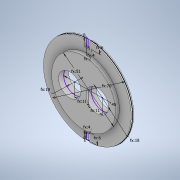
# Autodesk Inventor part: Spacer
Saved by Autodesk Inventor 2021.2 (Build 252289000, 289)
## iProperties
Created: 2023-01-29
Part Number: Spacer
Material: Типовые
Document SubType Name: Modeling
Designer: Andrei
Density: 1 g/cm^3
Appearance: По умолчанию
Author: Andrei
Autodesk Inventor part; units mm, degrees
ref_plane "YZ Plane" through (0, 0, 0) normal (1, 0, 0) x (0, 1, 0)
ref_plane "XZ Plane" through (0, 0, 0) normal (0, 1, 0) x (-1, 0, 0)
ref_plane "XY Plane" through (0, 0, 0) normal (0, 0, 1) x (1, 0, 0)
sketch "Эскиз1" plane through (0, 0, 0) normal (0, 0, 1) x (1, 0, 0)
  circle A0 centre (0, 0) radius 35
  circle A1 centre (0, 0) radius 25.5
  circle A2 centre (11, 0) radius 9
  circle A3 centre (-11, 0) radius 9
  line L0 (-2.0313, 35) -> (1.9687, 35)
  line L1 (1.9687, 35) -> (1.9687, 29)
  line L2 (1.9687, 29) -> (-2.0313, 29)
  line L3 (-2.0313, 29) -> (-2.0313, 35)
  line L4 (-2.0313, -29) -> (1.9687, -29)
  line L5 (1.9687, -29) -> (1.9687, -35)
  line L6 (1.9687, -35) -> (-2.0313, -35)
  line L7 (-2.0313, -35) -> (-2.0313, -29)
  line L8 (-0.0313, 25.5) -> (-0.0313, -25.5)
  line L9 (-0.0313, -25.5) -> (-0.0313, -35)
  line L10 (-0.0313, 35) -> (-0.0313, 25.5)
  point P0 (-2.0313, 25.419)
  point P1 (-2.0313, -25.419)
  point P2 (1.9687, -25.4239)
  point P3 (1.9687, 25.4239)
  point P4 (1.9687, -34.9446)
  point P5 (1.9687, 34.9446)
  point P6 (-2.0313, 34.941)
  point P7 (-2.0313, -34.941)
  dimension "d0" = 70
  dimension "d1" = 51
  dimension "d2" = 18
  dimension "d3" = 18
  dimension "d4" = 11
  dimension "d5" = 11
  dimension "d6" = 40
  dimension "d7" = 4
  dimension "d8" = 4
  dimension "d9" = 6
  dimension "d10" = 6
  dimension "d11" = 2
  dimension "d12" = 2
  dimension "d17" = 0
  dimension "d18" = 0
  constraints: 22 end point, 4 centre point, 4 parallel, 4 point on circle, 2 coincident, 2 horizontal, 2 perpendicular, 1 collinear, 1 point on line, 1 vertical
  measures "d0" diameter of A0
  measures "d1" diameter of A1
  measures "d2" diameter of A3
  measures "d3" diameter of A2
  measures "d4" distance of A2.centre point (0, 0)
  measures "d5" distance of A3.centre point (0, 0)
  measures "d7" distance of L1.end L2.end
  measures "d8" distance of L4.start L4.end
  measures "d9" distance of L0.end L1.end
  measures "d10" distance of L4.end L5.end
  measures "d11" distance between parallel lines of L7 L8
  measures "d12" distance between parallel lines of L3 L8
  measures "d17" distance from line of L10.start L0
  measures "d18" distance from line of L6 L9.end
extrude "Выдавливание1" add sketch "Эскиз1" along normal mid plane 8 contours L8 A1 | A1 L8
extrude "Выдавливание2" add sketch "Эскиз1" along normal mid plane 2 contours A0 L5 L4 L9 A1 L10 L2 L1 | L3 L2 L10 A1 L9 L4 L7 A0
equation "\"d0\" = dOuter"
equation "\"d1\" = dMount"
equation "\"d2\" = dHoles"
equation "\"d3\" = dHoles"
equation "\"d4\" = r2holes"
equation "\"d5\" = r2holes"
equation "\"d7\" = slotWidth"
equation "\"d8\" = slotWidth"
equation "\"d9\" = slotDepth"
equation "\"d10\" = slotDepth"
equation "\"d11\" = 0.5 * slotWidth"
equation "\"d12\" = 0.5 * slotWidth"
equation "\"dOuter\" = 70"
equation "\"dHoles\" = 18"
equation "\"hFlange\" = 4"
equation "\"hMount\" = 8"
equation "\"mountAngle\" = 60deg"
equation "\"dInternal\" = 44"
equation "\"dMount\" = 51"
equation "\"r2holes\" = 11"
equation "\"slotWidth\" = 4"
equation "\"slotDepth\" = 6"
